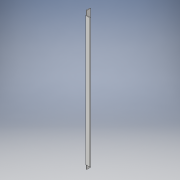
# Autodesk Inventor part: BumberMount.ver1-1111-2020
Saved by Autodesk Inventor 2018 (Build 220112000, 112)
## iProperties
Created: 2020-01-28
Part Number: BumberMount.ver1-1111-2020
Material: Generic
Document SubType Name: Modeling
Designer: JMHal
Density: 1 g/cm^3
Appearance: Default
Author: JMHal
Autodesk Inventor part; units mm, degrees
ref_plane "YZ Plane" through (0, 0, 0) normal (1, 0, 0) x (0, 1, 0)
ref_plane "XZ Plane" through (0, 0, 0) normal (0, 1, 0) x (-1, 0, 0)
ref_plane "XY Plane" through (0, 0, 0) normal (0, 0, 1) x (1, 0, 0)
sketch "Sketch1" plane through (0, 0, 0) normal (0, 1, 0) x (-1, 0, 0)
  line L0 (0, 0) -> (25.4, 0)
  line L1 (25.4, 0) -> (25.4, -25.4)
  line L2 (25.4, -25.4) -> (0, -25.4)
  line L3 (0, -25.4) -> (0, 0)
  line L4 (22.225, -22.225) -> (22.225, -3.175)
  line L5 (22.225, -3.175) -> (3.175, -3.175)
  line L6 (3.175, -3.175) -> (3.175, -22.225)
  line L7 (3.175, -22.225) -> (22.225, -22.225)
  line L8 (22.225, -22.225) -> (22.225, -25.4)
  line L9 (3.175, -3.175) -> (0, -3.175)
  dimension "d0" = 25.4
  dimension "d1" = 25.4
  dimension "d2" = 3.175
  constraints: 20 end point, 4 parallel, 4 perpendicular, 2 point on line, 1 horizontal, 3 other
  measures "d0" distance of L1.end L2.end
  measures "d1" distance of L0.end L1.end
  measures "d2" distance between parallel lines of L1 L4
extrude "Extrusion1" add sketch "Sketch1" along normal blind 814.3875 contours L0 L1 L2 L8 L4 L5 L9 L3
sketch "Sketch2" plane through (0, 0, -3.175) normal (0, 0, -1) x (-1, 0, 0)
  line L0 (0, 0) -> (22.225, 0) projected
  line L1 (22.225, 0) -> (22.225, 814.3875) projected
  line L2 (0, 814.3875) -> (22.225, 814.3875) projected
  line L3 (0, 0) -> (0, 814.3875) projected
  line L4 (22.225, 0) -> (22.225, 814.3875) projected
  line L5 (0, 0) -> (0, 814.3875) projected
  line L6 (22.225, 0) -> (0, 0)
  line L7 (0, 0) -> (0, 25.4)
  line L8 (0, 25.4) -> (22.225, 25.4)
  line L9 (22.225, 25.4) -> (22.225, 0)
  line L10 (0, 814.3875) -> (22.225, 814.3875)
  line L11 (22.225, 814.3875) -> (22.225, 788.9875)
  line L12 (22.225, 788.9875) -> (0, 788.9875)
  line L13 (0, 788.9875) -> (0, 814.3875)
  line L14 (0, 814.3875) -> (25.4, 814.3875)
  line L15 (25.4, 814.3875) -> (25.4, 788.9875)
  line L16 (25.4, 788.9875) -> (0, 788.9875)
  line L17 (0, 788.9875) -> (0, 814.3875)
  line L18 (25.4, 0) -> (25.4, 814.3875) projected
  line L19 (0, 25.4) -> (25.4, 25.4)
  line L20 (25.4, 25.4) -> (25.4, 0)
  line L21 (25.4, 0) -> (0, 0)
  line L22 (0, 0) -> (0, 25.4)
  dimension "d5" = 25.4
  dimension "d6" = 25.4
  constraints: 32 end point, 8 parallel, 4 horizontal, 4 perpendicular, 2 point on line, 1 collinear
  measures "d5" distance between parallel lines of L8 L0
  measures "d6" distance between parallel lines of L2 L12
extrude "Extrusion2" cut sketch "Sketch2" against normal blind 25.4 contours L3 L8 L1 L0 | L1 L19 L18 L21 | L3 L2 L1 L12 | L1 L14 L15 L16
body "Solid1"
